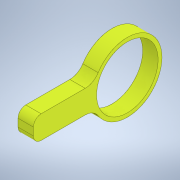
# Autodesk Inventor part: encoder_selector
Saved by Autodesk Inventor 2021 (Build 250183000, 183)
## iProperties
Created: 2021-12-13
Part Number: encoder_selector
Material: Generic
Document SubType Name: Modeling
Designer: Juan M. Casillas
Density: 1 g/cm^3
Appearance: Default
Author: Juan M. Casillas
## iProperties of the stored document _3DPrint.ipt
Created: 2021-12-13
Part Number: _3DPrint
Material: Generic
Document SubType Name: Modeling
Designer: Juan M. Casillas
Density: 1 g/cm^3
Appearance: Default
Author: Juan M. Casillas
Autodesk Inventor part; units mm, degrees
ref_plane "YZ Plane" through (0, 0, 0) normal (1, 0, 0) x (0, 1, 0)
ref_plane "XZ Plane" through (0, 0, 0) normal (0, 1, 0) x (-1, 0, 0)
ref_plane "XY Plane" through (0, 0, 0) normal (0, 0, 1) x (1, 0, 0)
sketch "Sketch1" plane through (0, 0, 0) normal (1, 0, 0) x (0, 1, 0)
  circle A0 centre (0, 0) radius 4
  arc A1 (-2.4231, 3.7919) -> (2.4231, 3.7919) centre (0, 0) ccw
  line L0 (-1.5, 11.2085) -> (-1.5, 5.4772)
  line L1 (1.5, 5.4772) -> (1.5, 11.2085)
  arc A2 (1.5, 5.4772) -> (2.4231, 3.7919) centre (3.5, 5.4772) ccw
  arc A3 (-2.4231, 3.7919) -> (-1.5, 5.4772) centre (-3.5, 5.4772) ccw
  line L2 (0.5, 12.2085) -> (-0.5, 12.2085)
  arc A4 (1.5, 11.2085) -> (0.5, 12.2085) centre (0.5, 11.2085) ccw
  arc A5 (-0.5, 12.2085) -> (-1.5, 11.2085) centre (-0.5, 11.2085) ccw
  point P0 (-1.5, 4.2426)
  point P1 (1.5, 4.2426)
  dimension "d0" = 8
  dimension "d1" = 9
  dimension "d4" = 2
  dimension "d8" = 1
  constraints: 12 point on circle, 8 tangent, 6 centre point, 6 end point, 2 coincident, 2 equal radius, 2 point on line, 1 parallel, 1 perpendicular
  measures "d0" diameter of A0
  measures "d1" diameter of A1
  measures "d4" radius of A2
  measures "d8" radius of A4
extrude "Extrusion1" add sketch "Sketch1" along normal blind 2
body "Solid1"
